nema-23 motor spacer_v1 (Autodesk Fusion 360 design; units mm, degrees)
Autodesk Fusion 360 part; units mm, degrees
sketch "Sketch1" plane through (0, 0, 0) normal (0, 0, 1) x (1, 0, 0)
  line L0 (-32.5, 32.5) -> (32.5, 32.5)
  line L1 (32.5, 32.5) -> (32.5, -32.5)
  line L2 (32.5, -32.5) -> (-32.5, -32.5)
  line L3 (-32.5, -32.5) -> (-32.5, 32.5)
  line L4 (-32.5, 32.5) -> (32.5, -32.5) construction
  line L5 (32.5, 32.5) -> (-32.5, -32.5) construction
  line L6 (-32.5, 0) -> (-32.5, 20) construction
  line L7 (-32.5, 20) -> (32.5, 20) construction
  line L8 (-32.5, 0) -> (-32.5, -20) construction
  line L9 (-32.5, -20) -> (32.5, -20) construction
  line L10 (-21, -22.75) -> (21, -22.75)
  arc A0 (21, -22.75) -> (21, -17.25) centre (21, -20) ccw
  line L11 (21, -17.25) -> (-21, -17.25)
  arc A1 (-21, -17.25) -> (-21, -22.75) centre (-21, -20) ccw
  line L12 (-21, -20) -> (21, -20) construction
  line L13 (-32.5, 0) -> (32.5, 0) construction
  line L14 (21, 17.25) -> (-21, 17.25)
  arc A2 (-21, 22.75) -> (-21, 17.25) centre (-21, 20) ccw
  line L15 (-21, 22.75) -> (21, 22.75)
  arc A3 (21, 17.25) -> (21, 22.75) centre (21, 20) ccw
  point P0 (0, -20)
  dimension "d1" = 65
  dimension "d2" = 65
  dimension "d3" = 5.5
  constraint horizontal L0
  constraint perpendicular L0 L1
  constraint parallel L0 L2
  constraint parallel L1 L3
  constraint coincident L4 origin
  constraint coincident L5 origin
  constraint midpoint L3 L6.start
  constraint coincident L3 L6.end
  constraint parallel L3 L6
  constraint coincident L1 L7.end
  constraint perpendicular L1 L7
  constraint coincident L3 L8.end
  constraint coincident L1 L9.end
  constraint perpendicular L1 L9
  constraint tangent L10 A0
  constraint tangent A0 L11
  constraint parallel L10 L11
  constraint tangent L11 A1
  constraint tangent L10 A1
  constraint parallel L9 L12
  constraint midpoint L9 P0
  constraint midpoint L12 P0
  constraint midpoint L1 L13.end
  constraint symmetric L10.start L13 A2.start
  constraint symmetric L10.end L13 L15.end
  constraint symmetric A0.end L13 L14.start
  constraint symmetric L11.end L13 L14.end
  constraint symmetric A0 L13 A3
  constraint symmetric A1 L13 A2
  measures "d1" distance of L1.end L2.end
  measures "d2" distance of L0.end L1.end
  measures "d3" diameter of A0
extrude "Extrude1" add sketch "Sketch1" along normal blind 0.8
fillet "Fillet1" radius 5.5 4 edges at (32.5, -32.5, 0.4) (32.5, 32.5, 0.4) (-32.5, 32.5, 0.4) (-32.5, -32.5, 0.4)
